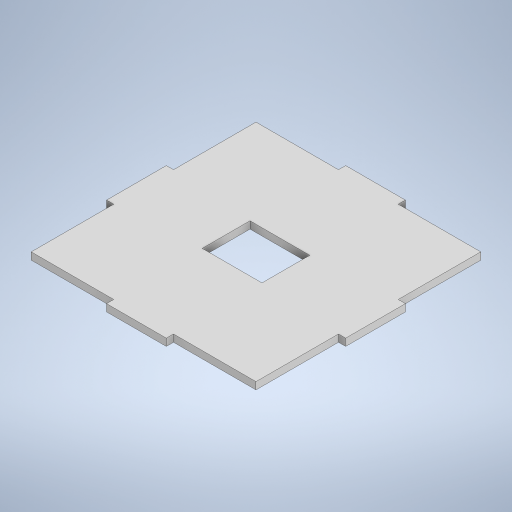
# Autodesk Inventor part: bolongan
Saved by Autodesk Inventor 2023 (Build 270158000, 158)
## iProperties
Created: 2023-02-07
Part Number: bolongan
Material: Generic
Document SubType Name: Modeling
Designer: Asus
Density: 1 g/cm^3
Appearance: Default
Author: Asus
Autodesk Inventor part; units mm, degrees
ref_plane "YZ Plane" through (0, 0, 0) normal (1, 0, 0) x (0, 1, 0)
ref_plane "XZ Plane" through (0, 0, 0) normal (0, 1, 0) x (-1, 0, 0)
ref_plane "XY Plane" through (0, 0, 0) normal (0, 0, 1) x (1, 0, 0)
sketch "Sketch1" plane through (0, 0, 0) normal (0, 1, 0) x (-1, 0, 0)
  line L0 (0, 0) -> (50, 0) construction
  line L1 (0, 0) -> (-50, 0) construction
  line L2 (0, 0) -> (0, 50) construction
  line L3 (0, 0) -> (0, -50) construction
  line L4 (0, -50) -> (12.5, -50)
  line L5 (12.5, -50) -> (12.5, -47)
  line L6 (12.5, -47) -> (47, -47)
  line L7 (47, -47) -> (47, -12.5)
  line L8 (47, -12.5) -> (50, -12.5)
  line L9 (50, -12.5) -> (50, 0)
  line L10 (50, 0) -> (50, 12.5)
  line L11 (50, 12.5) -> (47, 12.5)
  line L12 (47, 12.5) -> (47, 47)
  line L13 (47, 47) -> (12.5, 47)
  line L14 (12.5, 47) -> (12.5, 50)
  line L15 (12.5, 50) -> (-12.5, 50)
  line L16 (-12.5, 50) -> (-12.5, 47)
  line L17 (-12.5, 47) -> (-47, 47)
  line L18 (-47, 47) -> (-47, 12.5)
  line L19 (-47, 12.5) -> (-50, 12.5)
  line L20 (-50, 12.5) -> (-50, -12.5)
  line L21 (-50, -12.5) -> (-47, -12.5)
  line L22 (-47, -12.5) -> (-47, -47)
  line L23 (-47, -47) -> (-12.5, -47)
  line L24 (-12.5, -47) -> (-12.5, -50)
  line L25 (-12.5, -50) -> (0, -50)
  line L26 (0, 0) -> (0, 10) construction
  line L27 (0, 0) -> (0, -10)
  line L28 (0, 0) -> (12.5, 0) construction
  line L29 (12.5, 0) -> (12.5, -10)
  line L30 (12.5, -10) -> (-12.5, -10)
  line L31 (-12.5, -10) -> (-12.5, 10)
  line L32 (-12.5, 10) -> (12.5, 10)
  line L33 (12.5, 10) -> (12.5, 0)
  dimension "d0" = 50
  dimension "d1" = 50
  dimension "d2" = 50
  dimension "d3" = 50
  dimension "d4" = 12.5
  dimension "d5" = 3
  dimension "d6" = 34.5
  dimension "d7" = 34.5
  dimension "d8" = 3
  dimension "d9" = 12.5
  dimension "d10" = 3
  dimension "d11" = 34.5
  dimension "d12" = 34.5
  dimension "d13" = 3
  dimension "d14" = 25
  dimension "d15" = 3
  dimension "d16" = 34.5
  dimension "d17" = 34.5
  dimension "d18" = 3
  dimension "d19" = 25
  dimension "d20" = 3
  dimension "d21" = 34.5
  dimension "d22" = 34.5
  dimension "d23" = 3
  dimension "d24" = 10
  dimension "d25" = 10
  dimension "d26" = 12.5
  dimension "d27" = 10
  dimension "d28" = 25
  dimension "d29" = 20
  dimension "d30" = 25
  constraints: 68 end point, 16 perpendicular, 12 point on line, 3 vertical, 2 horizontal
  measures "d0" distance of L0.start L0.end
  measures "d1" distance of L0.start L1.end
  measures "d2" distance of L0.start L2.end
  measures "d3" distance of L0.start L3.end
  measures "d4" distance of L3.end L4.end
  measures "d5" distance of L4.end L5.end
  measures "d6" distance of L5.end L6.end
  measures "d7" distance of L6.end L7.end
  measures "d8" distance of L7.end L8.end
  measures "d9" distance of L0.end L10.end
  measures "d10" distance of L10.end L11.end
  measures "d11" distance of L11.end L12.end
  measures "d12" distance of L12.end L13.end
  measures "d13" distance of L13.end L14.end
  measures "d14" distance of L14.end L15.end
  measures "d15" distance of L15.end L16.end
  measures "d16" distance of L16.end L17.end
  measures "d17" distance of L17.end L18.end
  measures "d18" distance of L18.end L19.end
  measures "d19" distance of L19.end L20.end
  measures "d20" distance of L20.end L21.end
  measures "d21" distance of L21.end L22.end
  measures "d22" distance of L22.end L23.end
  measures "d23" distance of L23.end L24.end
  measures "d24" distance of L0.start L26.end
  measures "d25" distance of L0.start L27.end
  measures "d26" distance of L0.start L28.end
  measures "d27" distance of L28.end L29.end
  measures "d28" distance of L29.end L30.end
  measures "d29" distance of L30.end L31.end
  measures "d30" distance of L31.end L32.end
extrude "Extrusion1" add sketch "Sketch1" along normal blind 3
body "Solid1"
